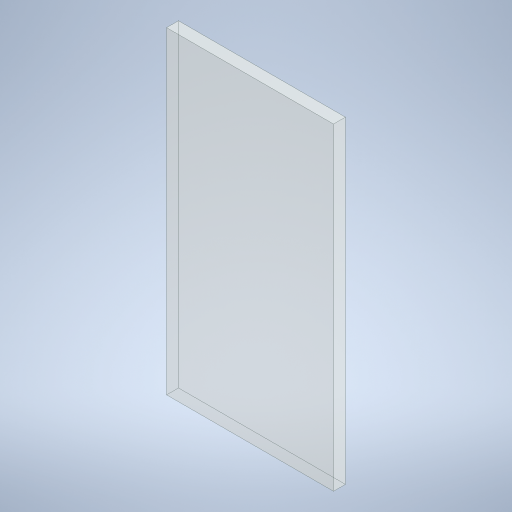
# Autodesk Inventor part: rapoukBottomPlexiv0
Saved by Autodesk Inventor 2024 (Build 280153000, 153)
## iProperties
Created: 2024-02-03
Part Number: rapoukBottomPlexiv0
Material: Všeobecné
Document SubType Name: Modeling
Designer: Roman Suk
Density: 1 g/cm^3
Appearance: Clear
MASSSFP: 400 g
SFP: 4HR
Author: Roman Suk
Autodesk Inventor part; units mm, degrees
ref_plane "YZ Plane" through (0, 0, 0) normal (1, 0, 0) x (0, 1, 0)
ref_plane "XZ Plane" through (0, 0, 0) normal (0, 1, 0) x (-1, 0, 0)
ref_plane "XY Plane" through (0, 0, 0) normal (0, 0, 1) x (1, 0, 0)
sketch "Sketch2" plane through (0, 0, 0) normal (0, 0, 1) x (1, 0, 0)
  line L0 (-21, -40) -> (21, -40)
  line L1 (21, -40) -> (21, 40)
  line L2 (21, 40) -> (-21, 40)
  line L3 (-21, 40) -> (-21, -40)
  line L4 (-21, -40) -> (21, 40) construction
  line L5 (21, -40) -> (-21, 40) construction
  point P0 (0, 0)
  dimension "d2" = 42
  dimension "d3" = 80
  constraints: 12 end point, 2 midpoint, 2 parallel, 1 horizontal, 1 perpendicular
  measures "d2" distance of L2.end L1.end
  measures "d3" distance of L1.end L0.end
extrude "Extrusion2" add sketch "Sketch2" along normal blind 3
body "Solid2"
